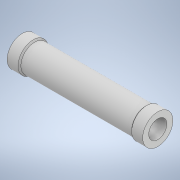
# Autodesk Inventor part: roller_ext
Saved by Autodesk Inventor 2021 (Build 250183000, 183)
## iProperties
Created: 2024-02-28
Part Number: roller_ext
Material: Generic
Document SubType Name: Modeling
Designer: Sebastián
Density: 1 g/cm^3
Appearance: Default
Author: Sebastián
Autodesk Inventor part; units mm, degrees
ref_plane "YZ Plane" through (0, 0, 0) normal (1, 0, 0) x (0, 1, 0)
ref_plane "XZ Plane" through (0, 0, 0) normal (0, 1, 0) x (-1, 0, 0)
ref_plane "XY Plane" through (0, 0, 0) normal (0, 0, 1) x (1, 0, 0)
sketch "Sketch1" plane through (0, 0, 0) normal (0, 1, 0) x (-1, 0, 0)
  line L0 (7.056, 3.3) -> (-24.7, 3.3)
  line L1 (-24.7, 3.3) -> (-24.7, 5.5)
  line L2 (-24.7, 5.5) -> (-20.7, 5.5)
  line L3 (-20.7, 5.5) -> (-20.2, 5)
  line L4 (-20.2, 5) -> (20.2, 5)
  line L5 (20.2, 5) -> (20.7, 5.5)
  line L6 (20.7, 5.5) -> (24.7, 5.5)
  line L7 (24.7, 5.5) -> (24.7, 3.3)
  line L8 (24.7, 3.3) -> (7.056, 3.3)
  line L9 (0, -1.1) -> (0, 6.6) construction
  line L10 (-34.58, 0) -> (34.58, 0) construction
  point P0 (0, 0)
  dimension "d0" = 3.3
  dimension "d1" = 40.4
  dimension "d2" = 49.4
  dimension "d3" = 0.5
  dimension "d4" = 5
  constraints: 18 end point, 5 perpendicular, 3 point on line, 3 symmetric about line, 1 horizontal, 1 parallel
  measures "d0" distance from line of L10 L7.end
  measures "d1" distance of L3.end L4.end
  measures "d2" distance of L1.end L6.end
  measures "d3" horizontal distance of L5.end L4.end
  measures "d4" vertical distance of point (0, 0) L4.end
revolve "Revolution1" add sketch "Sketch1" angle 360 about axis through (0, 0, 0) along (-1, 0, 0)
body "Solid1"
